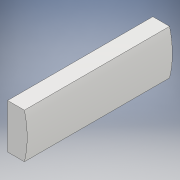
# Autodesk Inventor part: bepf_bateria_lipo
Saved by Autodesk Inventor 2017 (Build 210142000, 142)
## iProperties
Created: 2016-11-26
Part Number: bepf_bateria_lipo
Material: Tworzywo o ultrawysokiej masie cząsteczkowej, białe
Document SubType Name: Modeling
Designer: gagato
Density: 0.94 g/cm^3
Appearance: Gładki - biały
Mass: 81.4921 g
Surface Area: 156.877 cm^2
Volume: 86.6937 cm^3
Author: gagato
Autodesk Inventor part; units mm, degrees
ref_plane "YZ Plane" through (0, 0, 0) normal (1, 0, 0) x (0, 1, 0)
ref_plane "XZ Plane" through (0, 0, 0) normal (0, 1, 0) x (-1, 0, 0)
ref_plane "XY Plane" through (0, 0, 0) normal (0, 0, 1) x (1, 0, 0)
sketch "Szkic1" plane through (0, 0, 0) normal (1, 0, 0) x (0, 1, 0)
  line L0 (-65, 20) -> (65, 20)
  line L1 (65, 20) -> (65, -20)
  line L2 (65, -20) -> (-65, -20)
  line L3 (-65, -20) -> (-65, 20)
  line L4 (-65, 20) -> (65, -20) construction
  line L5 (65, 20) -> (-65, -20) construction
  point P0 (0, 0)
  dimension "d0" = 130
  dimension "d1" = 40
  constraints: 12 end point, 2 midpoint, 2 parallel, 1 horizontal, 1 perpendicular
  measures "d0" distance of L1.end L2.end
  measures "d1" distance of L0.end L1.end
extrude "Wyciągnięcie proste1" add sketch "Szkic1" along normal mid plane 15
sketch "Szkic2" plane through (-7.5, -65, -20) normal (0, -1, 0) x (1, 0, 0)
  line L0 (7.5, 20) -> (17.5, 20) construction
  line L1 (15, 0) -> (0, 0) construction
  arc A0 (15, 0) -> (15, 40) centre (-63.75, 20) ccw
  line L2 (15, 40) -> (15, 0) projected
  dimension "d4" = 10
  constraints: 3 point on circle, 2 end point, 1 centre point, 1 coincident, 1 horizontal
  measures "d4" distance of L0.start L0.end
extrude "Wyciągnięcie proste2" add sketch "Szkic2" against normal up to surface (130 mm away)
